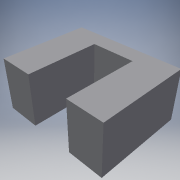
# Autodesk Inventor part: otackomer
Saved by Autodesk Inventor 2016 (Build 200138000, 138)
## iProperties
Created: 2017-01-08
Part Number: otackomer
Material: Generic
Document SubType Name: Modeling
Designer: Juraj
Density: 1 g/cm^3
Appearance: Default
Author: Juraj
Autodesk Inventor part; units mm, degrees
ref_plane "YZ Plane" through (0, 0, 0) normal (1, 0, 0) x (0, 1, 0)
ref_plane "XZ Plane" through (0, 0, 0) normal (0, 1, 0) x (-1, 0, 0)
ref_plane "XY Plane" through (0, 0, 0) normal (0, 0, 1) x (1, 0, 0)
sketch "Sketch1" plane through (0, 0, 0) normal (0, 0, 1) x (1, 0, 0)
  line L0 (-23.2184, 23.8212) -> (-10.2184, 23.8212)
  line L1 (-10.2184, 23.8212) -> (-10.2184, 17.8212)
  line L2 (-10.2184, 17.8212) -> (-23.2184, 17.8212)
  line L3 (-23.2184, 17.8212) -> (-23.2184, 23.8212)
  point P0 (0, 0)
  dimension "d0" = 13
  dimension "d1" = 6
  constraints: 8 end point, 2 parallel, 1 horizontal, 1 perpendicular
  measures "d0" distance of L1.end L2.end
  measures "d1" distance of L0.end L1.end
extrude "Extrusion1" add sketch "Sketch1" along normal blind 2
sketch "Sketch2" plane through (0, 0, 2) normal (0, 0, 1) x (1, 0, 0)
  line L0 (-23.2184, 17.8212) -> (-23.2184, 23.8212) projected
  line L1 (-23.2184, 23.8212) -> (-19.2184, 23.8212)
  line L2 (-19.2184, 23.8212) -> (-19.2184, 17.8212)
  line L3 (-19.2184, 17.8212) -> (-23.2184, 17.8212)
  line L4 (-23.2184, 17.8212) -> (-23.2184, 23.8212)
  line L5 (-23.2184, 17.8212) -> (-10.2184, 17.8212) projected
  line L6 (-10.2184, 23.8212) -> (-14.2184, 23.8212)
  line L7 (-14.2184, 23.8212) -> (-14.2184, 17.8212)
  line L8 (-14.2184, 17.8212) -> (-10.2184, 17.8212)
  line L9 (-10.2184, 17.8212) -> (-10.2184, 23.8212)
  line L10 (-10.2184, 17.8212) -> (-10.2184, 23.8212) projected
  point P0 (0, 0)
  dimension "d4" = 4
  dimension "d5" = 4
  dimension "d6" = 0
  constraints: 16 end point, 4 parallel, 2 horizontal, 2 perpendicular, 1 point on line
  measures "d4" distance of L2.end L3.end
  measures "d5" distance of L6.start L6.end
  measures "d6" distance between parallel lines of L9 L10
extrude "Extrusion2" add sketch "Sketch2" along normal blind 8.3
body "Solid1"
